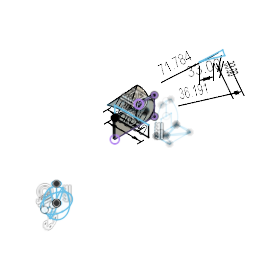
random testy kurz (Autodesk Fusion 360 design; units mm, degrees)
part number: 2025-10-18-17-38-49-562
Autodesk Fusion 360 part; units mm, degrees
box "BoxPrimitive1" add length 55 width 116.977 height 5 placed x (0, 0, -1) y (0, 1, 0) z (1, 0, 0) at (0, -81.9774, 107.7782) makes body 1
hole "Hole1" at (0, -20.9105, 106.0508) direction (1, 0, 0) diameter 20 depth 35 tip angle 118 bodies 1
sketch "1. 3d sketch" plane through (0, 0, 0) normal (1, 0, 0) x (0, 1, 0)
  line L0 (21.9857, 73.5147) -> (-37.7879, 98.0769)
  line L1 (-37.7879, 98.0769) -> (21.9857, 106.1497)
  line L2 (21.9857, 106.1497) -> (21.9857, 73.5147)
  line L3 (21.9857, 73.5147, 0) -> (21.9857, 73.5147, -70)
  line L4 (21.9857, 73.5147, -70) -> (-25.3321, 73.5147, -73.3997)
  line L5 (-25.3321, 73.5147, -73.3997) -> (-37.7879, 98.0769, 0)
  line L6 (-25.3321, 73.5147, -73.3997) -> (21.9857, 106.1497, 0)
  line L7 (21.9857, 73.5147, -70) -> (-0.7194, 90.4901, -35.2203)
  line L8 (21.9857, 73.5147, 0) -> (-34.2275, 91.0559, -20.9808)
  line L9 (-34.2275, 91.0559, -20.9808) -> (21.9857, 73.5147, -70)
  constraint vertical L2
revolve "Revolve1" add sketch "1. 3d sketch" angle 40 about axis through (-73.3997, -25.3321, 73.5147) along (0.936266, -0.158883, 0.313308) separate body contours L1 L5 L6 in plane through (-32.1901, -12.159, 90.0285) normal (-0.33399, -0.126157, 0.934096) makes body 2
sketch "Sketch5" plane through (5, 0, 0) normal (1, 0, 0) x (0, 1, 0)
  arc A0 (-30.7602, 107.7782) -> (-11.0608, 107.7782) centre (-20.9105, 106.0508) ccw
  line L0 (-30.7602, 107.7782) -> (-81.9774, 107.7782)
  line L1 (-81.9774, 107.7782) -> (-81.9774, 52.7782)
  line L2 (-81.9774, 52.7782) -> (34.9996, 52.7782)
  line L3 (34.9996, 52.7782) -> (34.9996, 107.7782)
  line L4 (34.9996, 107.7782) -> (-11.0608, 107.7782)
  line L5 (55, 0) -> (55, 36.4396)
  line L6 (55, 36.4396) -> (85, 36.4396)
  line L7 (85, 36.4396) -> (85, 0)
  line L8 (85, 0) -> (100, 0)
  line L9 (70, 36.4396) -> (70, 75)
  line L10 (55, 0) -> (40, 0)
  spline S0 degree 5 poles (55.7501, 72.2704) (53.739, 68.854) (49.965, 62.1845) (45.0486, 52.6705) (39.9886, 40.9694) (36.1769, 28.0086) (34.8788, 16.7467) (36.0455, 7.2187) (39.5476, -0.5482) (45.1408, -6.5443) (52.4296, -10.7894) (60.9084, -13.3156) (70, -14.153) (79.0916, -13.3156) (87.5704, -10.7894) (94.8592, -6.5443) (100.4524, -0.5482) (103.9545, 7.2187) (105.1212, 16.7467) (103.8231, 28.0086) (100.0114, 40.9694) (94.9514, 52.6705) (90.035, 62.1845) (86.261, 68.854) (84.2499, 72.2704) knots 0 0 0 0 0 0 0.05 0.1 0.15 0.2 0.25 0.3 0.35 0.4 0.45 0.5 0.55 0.6 0.65 0.7 0.75 0.8 0.85 0.9 0.95 1 1 1 1 1 1
  arc A1 (84.2499, 72.2704) -> (55.7501, 72.2704) centre (70, 36.4396) ccw
  spline S1 degree 5 poles (100, 0, 0) (100.4916, 0.2251, 3.1077) (101.3767, 0.6303, 9.0434) (102.4098, 1.1032, 17.1083) (103.1883, 1.4596, 26.1567) (103.0981, 1.4183, 34.4403) (101.8599, 0.8515, 39.4557) (99.3959, -0.2766, 40.9814) (95.693, -1.9717, 38.9807) (90.829, -4.1985, 33.6743) (84.9043, -6.9108, 25.3484) (79.3918, -9.4345, 16.4877) (74.8512, -11.5132, 8.686) (71.6467, -12.9802, 2.9796) (70, -13.734, 0) knots 0 0 0 0 0 0 0.1 0.2 0.3 0.4 0.5 0.6 0.7 0.8 0.9 1 1 1 1 1 1
  line L11 (40, 0, 0) -> (100, 0, 40)
  spline S2 degree 5 poles (40, 0, 0) (39.5084, 0.2251, 3.1077) (38.6233, 0.6303, 9.0434) (37.5902, 1.1032, 17.1083) (36.8117, 1.4596, 26.1567) (36.9019, 1.4183, 34.4403) (38.1401, 0.8515, 39.4557) (40.6041, -0.2766, 40.9814) (44.307, -1.9717, 38.9807) (49.171, -4.1985, 33.6743) (55.0957, -6.9108, 25.3484) (60.6082, -9.4345, 16.4877) (65.1488, -11.5132, 8.686) (68.3533, -12.9802, 2.9796) (70, -13.734, 0) knots 0 0 0 0 0 0 0.1 0.2 0.3 0.4 0.5 0.6 0.7 0.8 0.9 1 1 1 1 1 1
  line L12 (40, 0, 40) -> (100, 0, 40)
  line L13 (40, 0) -> (70, -13.734)
  line L14 (70, -13.734) -> (100, 0)
  line L15 (40, 0, 40) -> (40, 0, 0)
  line L16 (100, 0, 40) -> (100, 0, 0)
  line L17 (40, 0) -> (100, 0)
  point P0 (70, -13.734)
  point P1 (100, 0)
  point P2 (40, 0)
  constraint perpendicular L2 L5
  constraint perpendicular L5 L6
  constraint perpendicular L2 L7
  constraint perpendicular L7 L8
  constraint midpoint L6 L9.start
  constraint perpendicular L6 L9
  constraint symmetric L7.end L9 L5.start
  constraint symmetric P1 L9 P2
  constraint coincident P1 L8.end
  constraint coincident P0 L13.end
  constraint coincident P2 L10.end
sketch "pokus o sroubovici" plane through (5, 0, 0) normal (1, 0, 0) x (0, 1, 0)
  line L0 (-81.9774, 107.7782, 0) -> (-81.9774, 107.7782, 100)
  line L1 (-81.9774, 107.7782, 100) -> (-81.9774, 140, 100)
  line L2 (-81.9774, 140, 100) -> (-81.9774, 140, 0)
  line L3 (-81.9774, 140) -> (-81.9774, 107.7782)
  line L4 (168.5659, 125.9979, 0) -> (199.5986, 125.9704, 11.2235)
  line L5 (199.5986, 125.9704, 11.2235) -> (202.2471, 146.0456, 41.2191)
  line L6 (202.2471, 146.0456, 41.2191) -> (186.3934, 173.2955, 50.9713)
  line L7 (186.3934, 173.2955, 50.9713) -> (168.5659, 125.9979, 0)
  circle A0 through (-288.9345, 0, 24.4036) (-273.9345, 0, 33.0639) (-273.9345, 0, 15.7434)
  line L8 (-288.92, 0, 23.8658) -> (-313.92, 0, 23.8658)
  circle A1 through (-313.9345, 0, 24.4036) (-261.4345, -26.25, 39.5591) (-261.4345, 26.25, 9.2482)
  line L9 (-279.2455, 0, 14.4084) -> (-282.5207, 30.1514, 6.9957)
  line L10 (-278.9345, 0, 24.4036) -> (-278.9345, 50, 24.4036)
  circle A2 through (-288.9345, 50, 24.4036) (-273.9345, 50, 33.0639) (-273.9345, 50, 15.7434)
  circle A3 through (-261.4345, -30.3109, 24.4036) (-264.9513, 28.2804, 39.5591) (-310.4177, 2.0304, 9.2482)
  circle A4 through (-261.4345, 30.3109, 24.4036) (-310.4177, -2.0304, 39.5591) (-264.9513, -28.2804, 9.2482)
  line L11 (-81.9774, 52.7782) -> (34.9996, 52.7782)
  line L12 (34.9996, 52.7782) -> (34.9996, 107.7782)
  line L13 (34.9996, 107.7782) -> (-11.0608, 107.7782)
  circle A5 centre (7.4996, 80.2782) radius 27.5
  point P0 (-81.9774, 107.7782)
  dimension "d10" = 100
  dimension "d11" = 100
  dimension "d12" = 33
  dimension "d13" = 33
  dimension "d14" = 71.7841
  dimension "d15" = 36.1907
  dimension "d17" = 360
  constraint coincident P0 L3.end
  constraint tangent L11 A5
  constraint tangent L12 A5
  constraint tangent L13 A5
  measures "d10" distance of P0 L3.end
